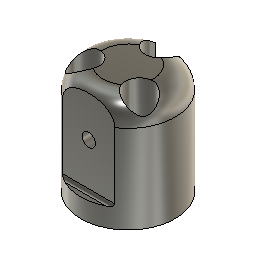
Epaule_4 (Autodesk Fusion 360 design; units mm, degrees)
Autodesk Fusion 360 part; units mm, degrees
note: some values were not read from the file. Set by a fixed rule: which sketch regions a step uses.
sketch "Sketch1" plane through (0, 0, 0) normal (0, 0, 1) x (1, 0, 0)
  circle A0 centre (0, 0) radius 3.5
  circle A1 centre (0, 0) radius 10 construction
  circle A2 centre (0, 10) radius 2.1
  line L0 (0, 10) -> (0, 0) construction
  circle A3 centre (-8.6603, -5) radius 2.1
  circle A4 centre (8.6603, -5) radius 2.1
  line L1 (0, 0) -> (0, -10) construction
  line L2 (1.6, -3.1129) -> (1.6, -10)
  line L3 (1.6, -10) -> (-1.6, -10)
  line L4 (-1.6, -10) -> (-1.6, -3.1129)
  circle A5 centre (0, 0) radius 15
  circle A6 centre (8.6603, -5) radius 4.5
  circle A7 centre (0, 10) radius 4.5
  circle A8 centre (-8.6603, -5) radius 4.5
  line L5 (-8.2916, -12.5) -> (8.2916, -12.5)
  line L6 (-8.2916, 12.5) -> (8.2916, 12.5)
  dimension "d1" = 7
  dimension "d2" = 20
  dimension "d3" = 4.2
  dimension "d5" = 360
  dimension "d6" = 10
  dimension "d7" = 3.2
  dimension "d8" = 30
  dimension "d20" = 9
  dimension "d21" = 9
  dimension "d22" = 9
  dimension "d33" = 12.5
  dimension "d50" = 12.5
  constraint coincident A0.centre A1.centre
  constraint concentric A0 A1
  constraint coincident A1 A2.centre
  constraint coincident A2.centre L0.start
  constraint vertical L0
  constraint parallel L0 L1
  constraint coincident A0 L2.start
  constraint parallel L0 L2
  constraint coincident A0 L4.end
  constraint perpendicular L3 L4
  constraint midpoint L1.end L3
  constraint horizontal L3
  constraint concentric A4 A6
  constraint concentric A2 A7
  constraint concentric A3 A8
  constraint coincident A5 L5.start
  constraint coincident A5 L5.end
  constraint horizontal L5
  constraint coincident A5 L6.start
  constraint coincident A5 L6.end
  constraint horizontal L6
  measures "d1" diameter of A0
  measures "d2" diameter of A1
  measures "d3" diameter of A2
  measures "d6" distance of A0.centre L1.end
  measures "d7" distance of L2.end L3.end
  measures "d8" diameter of A5
  measures "d20" diameter of A6
  measures "d21" diameter of A7
  measures "d22" diameter of A8
  measures "d33" vertical distance of A0.centre L5.end
  measures "d50" vertical distance of A0.centre L6.end
extrude "Extrude4" add sketch "Sketch1" along normal blind 35 contours A0 | A0 L2 L3 L4 | A5 A7 L5 L6 | A5 A7 L6 | A5 L5 | A7 L6 | A7 L6 | A6 | A8
extrude "Extrude7" cut sketch "Sketch1" along normal through all from surface at 5 contours A7 L6 | A7 L6 | A6 | A8
extrude "Extrude8" cut sketch "Sketch1" along normal through all from surface at 6 contours A5 A7 L6 | A5 L5 | A7 L6 picked at (0.3332, 13.3485)
sketch "Sketch6" plane through (0, -12.5, 0) normal (0, -1, 0) x (1, 0, 0)
  line L0 (-8.2916, 35) -> (-8.2916, 6)
  circle A0 centre (0, 20.5) radius 2.1
  circle A1 centre (0, 20.5) radius 4.25
  line L1 (8.2916, 35) -> (-8.2916, 35)
  line L2 (-8.2916, 6) -> (8.2916, 6)
  line L3 (8.2916, 6) -> (8.2916, 35)
  line L4 (8.2916, 35) -> (-8.2916, 6) construction
  dimension "d40" = 4.2
  dimension "d44" = 8.5
  constraint concentric A0 A1
  constraint coincident L1.start L3.end
  constraint coincident L0.end L2.start
  constraint midpoint A0.centre L4
  measures "d40" diameter of A0
  measures "d44" diameter of A1
fillet "Fillet1" radius 1 1 edges at (0, -12.5, 6)
fillet "Fillet2" radius 7 2 edges at (15, 0, 35) (-15, 0, 35)
extrude "Extrude9" cut sketch "Sketch6" against normal through all contours A0
named bodies: "Epaule_4"
